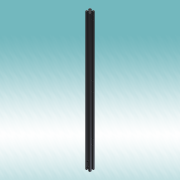
# Autodesk Inventor part: HFSB5-2020-550-LCH-RWV-AH30-BH240-CH280-DH442-EH462
Saved by Autodesk Inventor 2015 (Build 190159000, 159)
## iProperties
Category: PARTsolutions
Company: MISUMI
Created: 2016-02-28
Part Number: HFSB5-2020-550-LCH-RWV-AH30-BH240-CH280-DH442-EH462
Catalog Web Link: www.cadenas.de
Description: NFS5-2020, NFSB5-2020, HFS5-2020, HFSB5-2020, CAF5-2020, HFSY5-2020, NFSF5-2020, HFSF5-2020, HFSFB5-2020, NFST5-2020, HFST5-2020, HFSTB5-2020, HFSH5-2020, HFSC5-2020-HFS5 Series Aluminum Extrusions 20 Square -1 Slot-
Vendor: MISUMI
Document SubType Name: Modeling
Designer: psAdmin
Manufacturer: MISUMI
Mass: 98.1163 g
Surface Area: 954.349 cm^2
Volume: 98.1163 cm^3
Density: 1 g/cm^3
Material: 一般
Appearance: PSOLRGB-175-175-175
PSOL_IDENT_0: {$CADENAS_DATA\23d-libs\misumi\metric\38_al_extrusions_blackets\5\hfs5_2020.prj},646 {VTYP=3D},{NB=H
PSOL_IDENT_1: FSB5-2020-550-LCH-RWV-AH30-BH240-CH280-DH442-EH462},{LINA=HFSB5-2020-550-LCH-RWV-AH30-BH240-CH280-DH
PSOL_IDENT_2: 442-EH462},{NN=NFS5-2020, NFSB5-2020, HFS5-2020, HFSB5-2020, CAF5-2020, HFSY5-2020, NFSF5-2020, HFSF
PSOL_IDENT_3: 5-2020, HFSFB5-2020, NFST5-2020, HFST5-2020, HFSTB5-2020, HFSH5-2020, HFSC5-2020},{DATE=17.07.2015 1
PSOL_IDENT_4: 0:47:07},{GEOMDATE=28.10.2014 00:00:00},{VERSION=},{LINEID=140},{LINESUBID=-1},{WBVAR=L,ALT1,ALT2,AL
PSOL_IDENT_5: T4,ALT5,CP5,DL5,DR5,ALT6,ALT9,ALT10,ALT11,HP6,NHL6,DL6,NHR6,DR6,ALT7,ALT8,NH9,AH,BH,CH,DH,EH,NH10,AV
PSOL_IDENT_6: ,BV,CV,DV,EV,NH11,AP,BP,CP,DP,EP,ALT12,ALT13,Z,NH12,XA,XB,XC,XD,XE,NH13,YA,YB,YC,YD,YE,ALT16,HP16,DL
PSOL_IDENT_7: 16,DR16,ALT17,HQ17,JLP,ALT20}  {NB=HFSB5-2020-550-LCH-RWV-AH30-BH240-CH280-DH442-EH462},{LINA=HFSB5-
PSOL_IDENT_8: 2020-550-LCH-RWV-AH30-BH240-CH280-DH442-EH462},{KT=DUMMY},{PN=HFSB5-2020-550-LCH-RWV-AH30-BH240-CH28
PSOL_IDENT_9: 0-DH442-EH462},{TPS=HFSB5-2020},{MAT=A6N01SS-T5 Aluminum Alloy or 6005A-T5 Aluminum Alloy},{ST=Black
PSOL_IDENT_10: Anodize},{FRMW=20},{FRMH=20},{FRD=4.2},{L=550},{MASS=0.5},{SA=183},{LX=0.742x10^4},{LY=0.742x10^4},
PSOL_IDENT_11: {ALT1=},{M1=0},{DPL1=0},{DPR1=0},{ALT1PN=},{ALT2=},{ALT2ALG= '','w/o End Tapping (Heli-Coil Insert)'
PSOL_IDENT_12: ,'LHP','with LHP (Tapping on the Left (Heli-Coil Insert))','RHP','with RHP (Tapping on the Right (He
PSOL_IDENT_13: li-Coil Insert))','HPW','with HPW (Tapping on Both Ends (Heli-Coil Insert))' },{M2=0},{DP2=0},{ALT2P
PSOL_IDENT_14: N=},{ALT4=},{ALT4ALG= '', 'w/o SC (High Precision Cut)', 'SC', 'with SC (High Precision Cut)' },{ALT
PSOL_IDENT_15: 4PN=},{ALT5=},{ALT5ALG= '','w/o 45 Degree Cut','1','with 45 Degree Cut' },{CP5=},{CP5ALG= '','N/A' }
PSOL_IDENT_16: ,{DL5=},{DL5ALG= '','N/A' },{DR5=},{DR5ALG= '','N/A' },{FRMLALT5=0},{FRMRALT5=0},{ALT5PN=},{ALT6=1},
PSOL_IDENT_17: {ALT6ALG= '','w/o Fastening Location Wrench Access Hole Alterations','1','with Fastening Location Wr
PSOL_IDENT_18: ench Access Hole Alterations' },{ALT9=1},{ALT9ALG= '','w/o Location Specified Wrench Access Hole Alt
PSOL_IDENT_19: eratons (Horizontal)','1','with Location Specified Wrench Access Hole Alteratons (Horizontal)' },{AL
PSOL_IDENT_20: T10=},{ALT10ALG= '','w/o Location Specified Wrench Access Hole Alteratons (Vertical)','1','with Loca
PSOL_IDENT_21: tion Specified Wrench Access Hole Alteratons (Vertical)' },{ALT11=},{ALT11ALG= '','w/o Location Spec
PSOL_IDENT_22: ified Wrench Access Hole Alteratons (Crisscross)','1','with Location Specified Wrench Access Hole Al
PSOL_IDENT_23: teratons (Crisscross)' },{HP6=LR},{HP6ALG= 'L','Left','R','Right','LR','Both Sides' },{NHL6=C},{NHL6
PSOL_IDENT_24: ALG= 'C','C (Wrench Holes in Single Line)','W','W (Wrench Holes in Two Lines)','E','E (Wrench Holes
PSOL_IDENT_25: in Three Lines)' },{DL6=H},{DL6ALG= 'H','H (Horizontal)','V','V (Vertical)','P','P (Crisscross)' },{
PSOL_IDENT_26: NHR6=W},{NHR6ALG= 'C','C (Wrench Holes in Single Line)','W','W (Wrench Holes in Two Lines)','E','E (
PSOL_IDENT_27: Wrench Holes in Three Lines)' },{DR6=V},{DR6ALG= 'H','H (Horizontal)','V','V (Vertical)','P','P (Cri
PSOL_IDENT_28: sscross)' },{HL6=10},{HL6D=10},{HR6=10},{HR6D=10},{J6=20},{J6D=20},{K6=20},{K6D=0},{DD6=7.35},{DD6AL
PSOL_IDENT_29: G=7.35},{ALT7=},{ALT7ALG= '','w/o FL (Shifts The Wrench Hole on The Left Side 3mm Toward The Left En
PSOL_IDENT_30: d)','FL','with FL (Shifts The Wrench Hole on The Left Side 3mm Toward The Left End)' },{ALT8=},{ALT8
PSOL_IDENT_31: ALG= '','w/o FR (Shifts The Wrench Hole on The Right Side 3mm Toward The Right End)','FR','with FR (
PSOL_IDENT_32: Shifts The Wrench Hole on The Right Side 3mm Toward The Right End)' },{ALT678PN=-LCH-RWV},{NH9=5},{N
PSOL_IDENT_33: H9MAX=5},{NH9ALG=[1:5/1]},{AH=30.0},{AHMIN=7},{AHMAX=505},{AHALG=[7:505/0.5]},{BH=240.0},{BHMIN=39.5
PSOL_IDENT_34: },{BHMAX=514.5},{BHALG=[39.5:514.5/0.5]},{CH=280.0},{CHMIN=249.5},{CHMAX=524},{CHALG=[249.5:524/0.5]
PSOL_IDENT_35: },{DH=442.0},{DHMIN=289.5},{DHMAX=533.5},{DHALG=[289.5:533.5/0.5]},{EH=462.0},{EHMIN=451.5},{EHMAX=5
PSOL_IDENT_36: 43},{EHALG=[451.5:543/0.5]},{NH10=0},{NH10MAX=5},{NH10ALG=[0]},{AV=0.0},{AVMIN=7},{AVMAX=552.5},{AVA
PSOL_IDENT_37: LG=[0]},{BV=0.0},{BVMIN=9.5},{BVMAX=562},{BVALG=[0]},{CV=0.0},{CVMIN=9.5},{CVMAX=571.5},{CVALG=[0]},
PSOL_IDENT_38: {DV=0.0},{DVMIN=9.5},{DVMAX=581},{DVALG=[0]},{EV=0.0},{EVMIN=9.5},{EVMAX=543},{EVALG=[0]},{NH11=0},{
PSOL_IDENT_39: NH11MAX=5},{NH11ALG=[0]},{AP=0.0},{APMIN=7},{APMAX=552.5},{APALG=[0]},{BP=0.0},{BPMIN=9.5},{BPMAX=56
PSOL_IDENT_40: 2},{BPALG=[0]},{CP=0.0},{CPMIN=9.5},{CPMAX=571.5},{CPALG=[0]},{DP=0.0},{DPMIN=9.5},{DPMAX=581},{DPAL
PSOL_IDENT_41: G=[0]},{EP=0.0},{EPMIN=9.5},{EPMAX=543},{EPALG=[0]},{ALT9PN=-AH30-BH240-CH280-DH442-EH462},{ALT10PN=
PSOL_IDENT_42: },{ALT11PN=},{ALT91011PN=-AH30-BH240-CH280-DH442-EH462},{ALT12=},{ALT12ALG= '','w/o Counterbore Hole
PSOL_IDENT_43: in Specified Position (Vertical)','1','with Counterbore Hole in Specified Position (Vertical)' },{A
PSOL_IDENT_44: LT13=},{ALT13ALG= '','w/o Counterbore Hole in Specified Position (Horizontal)','1','with Counterbore
PSOL_IDENT_45: Hole in Specified Position (Horizontal)' },{Z=},{ZALG= '','N/A' },{DD12=0.0},{DD112=0.0},{NH12=0},{
PSOL_IDENT_46: NH12MAX=5},{NH12ALG=[0]},{XA=0.0},{XAMIN=7},{XAMAX=545},{XAALG=[0]},{XB=0.0},{XBMIN=2},{XBMAX=547},{
PSOL_IDENT_47: XBALG=[0]},{XC=0.0},{XCMIN=2},{XCMAX=549},{XCALG=[0]},{XD=0.0},{XDMIN=2},{XDMAX=551},{XDALG=[0]},{XE=
PSOL_IDENT_48: 0.0},{XEMIN=2},{XEMAX=543},{XEALG=[0]},{NH13=0},{NH13MAX=5},{NH13ALG=[0]},{YA=0.0},{YAMIN=7},{YAMAX=
PSOL_IDENT_49: 545},{YAALG=[0]},{YB=0.0},{YBMIN=2},{YBMAX=547},{YBALG=[0]},{YC=0.0},{YCMIN=2},{YCMAX=549},{YCALG=[0
PSOL_IDENT_50: ]},{YD=0.0},{YDMIN=2},{YDMAX=551},{YDALG=[0]},{YE=0.0},{YEMIN=2},{YEMAX=543},{YEALG=[0]},{ALT12PN=},
PSOL_IDENT_51: {ALT13PN=},{ALT1213PN=},{ALT16=},{ALT16ALG= '','w/o M Type Hole Alteration','1','with M Type Hole Al
PSOL_IDENT_52: teration' },{HP16=},{HP16ALG= '','N/A' },{DL16=},{DL16ALG= '','N/A' },{DR16=},{DR16ALG= '','N/A' },{
PSOL_IDENT_53: H116=0},{D16=0.0},{ALT16PN=},{ALT17=},{ALT17ALG= '','w/o L Type Hole Alteration (Top)','1','with L T
PSOL_IDENT_54: ype Hole Alteration (Top)' },{HQ17=0},{HQ17ALG=0},{JLP=0},{JLPMIN=4.9},{JLPMAX=0},{JLPALG=[0]},{L17=
PSOL_IDENT_55: 0},{D17=0.0},{ALT17PN=},{ALT20=},{ALT20PN=},{ERRORALT01=OK},{ERRORALT02=OK},{ERRORALT05=OK},{ERRORAL
PSOL_IDENT_56: T06091=OK},{ERRORALT06092=OK},{ERRORALT06093=OK},{ERRORALT06094=OK},{ERRORALT06101=OK},{ERRORALT0610
PSOL_IDENT_57: 2=OK},{ERRORALT06103=OK},{ERRORALT06104=OK},{ERRORALT06111=OK},{ERRORALT06112=OK},{ERRORALT06113=OK}
PSOL_IDENT_58: ,{ERRORALT06114=OK},{ERRORALT06121=OK},{ERRORALT06122=OK},{ERRORALT06123=OK},{ERRORALT06124=OK},{ERR
PSOL_IDENT_59: ORALT06131=OK},{ERRORALT06132=OK},{ERRORALT06133=OK},{ERRORALT06134=OK},{ERRORALT0616=OK},{ERRORALT0
PSOL_IDENT_60: 6171=OK},{ERRORALT06172=OK},{ERRORALT06173=OK},{ERRORALT0911=OK},{ERRORALT0913=OK},{ERRORALT0916=OK}
PSOL_IDENT_61: ,{ERRORALT0917=OK},{ERRORALT1011=OK},{ERRORALT1012=OK},{ERRORALT1016=OK},{ERRORALT1017=OK},{ERRORALT
PSOL_IDENT_62: 1112=OK},{ERRORALT1113=OK},{ERRORALT1116=OK},{ERRORALT1117=OK},{ERRORALT1216=OK},{ERRORALT1217=OK},{
PSOL_IDENT_63: ERRORALT1316=OK},{ERRORALT1317=OK},{ERRORALT1617=OK},{ERRORPN=},{TFW=0}
NN: NFS5-2020, NFSB5-2020, HFS5-2020, HFSB5-2020, CAF5-2020, HFSY5-2020, NFSF5-2020, HFSF5-2020, HFSFB5-2020, NFST5-2020, HFST5-2020, HFSTB5-2020, HFSH5-2020, HFSC5-2020
NT: HFS5 Series Aluminum Extrusions 20 Square -1 Slot-
NB: HFSB5-2020-550-LCH-RWV-AH30-BH240-CH280-DH442-EH462
NBSYN: $PN.
LINA: HFSB5-2020-550-LCH-RWV-AH30-BH240-CH280-DH442-EH462
PN: HFSB5-2020-550-LCH-RWV-AH30-BH240-CH280-DH442-EH462
TPS: HFSB5-2020
MAT: A6N01SS-T5 Aluminum Alloy or 6005A-T5 Aluminum Alloy
ST: Black Anodize
L: 550
MASS: 0.5
SA: 183
LX: 0.742x10^4
LY: 0.742x10^4
ALT1: w/o End Tapping
M1: 0
DPL1: 0
DPR1: 0
ALT2: w/o End Tapping (Heli-Coil Insert)
M2: 0
DP2: 0
ALT4: w/o SC (High Precision Cut)
ALT5: w/o 45 Degree Cut
CP5: N/A
DL5: N/A
DR5: N/A
ALT6: with Fastening Location Wrench Access Hole Alterations
ALT9: with Location Specified Wrench Access Hole Alteratons (Horizontal)
ALT10: w/o Location Specified Wrench Access Hole Alteratons (Vertical)
ALT11: w/o Location Specified Wrench Access Hole Alteratons (Crisscross)
HP6: Both Sides
NHL6: C (Wrench Holes in Single Line)
DL6: H (Horizontal)
NHR6: W (Wrench Holes in Two Lines)
DR6: V (Vertical)
HL6D: 10
HR6D: 10
J6D: 20
K6D: 0
DD6: 7.35
ALT7: w/o FL (Shifts The Wrench Hole on The Left Side 3mm Toward The Left End)
ALT8: w/o FR (Shifts The Wrench Hole on The Right Side 3mm Toward The Right End)
NH9: 5
AH: 30.0
BH: 240.0
CH: 280.0
DH: 442.0
EH: 462.0
NH10: 0
AV: 0.0
BV: 0.0
CV: 0.0
DV: 0.0
EV: 0.0
NH11: 0
AP: 0.0
BP: 0.0
CP: 0.0
DP: 0.0
EP: 0.0
ALT12: w/o Counterbore Hole in Specified Position (Vertical)
ALT13: w/o Counterbore Hole in Specified Position (Horizontal)
Z: N/A
DD12: 0.0
DD112: 0.0
NH12: 0
XA: 0.0
XB: 0.0
XC: 0.0
XD: 0.0
XE: 0.0
NH13: 0
YA: 0.0
YB: 0.0
YC: 0.0
YD: 0.0
YE: 0.0
ALT16: w/o M Type Hole Alteration
HP16: N/A
DL16: N/A
DR16: N/A
H116: 0
D16: 0.0
ALT17: w/o L Type Hole Alteration (Top)
HQ17: 0
JLP: 0
D17: 0.0
ALT20: w/o CW (End Face C Chamfering)
SUPPLIER: MISUMI
ARTICLENO: HFSB5-2020-550-LCH-RWV-AH30-BH240-CH280-DH442-EH462
BOMINFO: HFSB5-2020-550-LCH-RWV-AH30-BH240-CH280-DH442-EH462
CREATOR: CADENAS GmbH
Title: HFSB5-2020-550-LCH-RWV-AH30-BH240-CH280-DH442-EH462
Author: Cadenas PARTsolutions
Comments: HFS5 Series Aluminum Extrusions 20 Square -1 Slot-
Autodesk Inventor part; units mm, degrees
sketch "Sketch_1" plane through (0, 0, 0) normal (0, 0, 1) x (1, 0, 0)
  line L0 (-10, 3) -> (-8, 3)
  line L1 (-8, 3) -> (-8, 6)
  line L2 (-8, 6) -> (-7.0607, 6)
  line L3 (-7.0607, 6) -> (-4, 2.9393)
  line L4 (-4, 2.9393) -> (-4, 0.5196)
  line L5 (-4, 0.5196) -> (-3.7, 0)
  line L6 (-3.7, 0) -> (-4, -0.5196)
  line L7 (-4, -0.5196) -> (-4, -2.9393)
  line L8 (-4, -2.9393) -> (-7.0607, -6)
  line L9 (-7.0607, -6) -> (-8, -6)
  line L10 (-8, -6) -> (-8, -3)
  line L11 (-8, -3) -> (-10, -3)
  line L12 (-10, -3) -> (-10, -9)
  arc A0 (-10, -9) -> (-9, -10) centre (-9, -9) ccw
  line L13 (-9, -10) -> (-3, -10)
  line L14 (-3, -10) -> (-3, -8)
  line L15 (-3, -8) -> (-6, -8)
  line L16 (-6, -8) -> (-6, -7.0607)
  line L17 (-6, -7.0607) -> (-2.9393, -4)
  line L18 (-2.9393, -4) -> (-0.5196, -4)
  line L19 (-0.5196, -4) -> (0, -3.7)
  line L20 (0, -3.7) -> (0.5196, -4)
  line L21 (0.5196, -4) -> (2.9393, -4)
  line L22 (2.9393, -4) -> (6, -7.0607)
  line L23 (6, -7.0607) -> (6, -8)
  line L24 (6, -8) -> (3, -8)
  line L25 (3, -8) -> (3, -10)
  line L26 (3, -10) -> (9, -10)
  arc A1 (9, -10) -> (10, -9) centre (9, -9) ccw
  line L27 (10, -9) -> (10, -3)
  line L28 (10, -3) -> (8, -3)
  line L29 (8, -3) -> (8, -6)
  line L30 (8, -6) -> (7.0607, -6)
  line L31 (7.0607, -6) -> (4, -2.9393)
  line L32 (4, -2.9393) -> (4, -0.5196)
  line L33 (4, -0.5196) -> (3.7, 0)
  line L34 (3.7, 0) -> (4, 0.5196)
  line L35 (4, 0.5196) -> (4, 2.9393)
  line L36 (4, 2.9393) -> (7.0607, 6)
  line L37 (7.0607, 6) -> (8, 6)
  line L38 (8, 6) -> (8, 3)
  line L39 (8, 3) -> (10, 3)
  line L40 (10, 3) -> (10, 9)
  arc A2 (10, 9) -> (9, 10) centre (9, 9) ccw
  line L41 (9, 10) -> (3, 10)
  line L42 (3, 10) -> (3, 8)
  line L43 (3, 8) -> (6, 8)
  line L44 (6, 8) -> (6, 7.0607)
  line L45 (6, 7.0607) -> (2.9393, 4)
  line L46 (2.9393, 4) -> (0.5196, 4)
  line L47 (0.5196, 4) -> (0, 3.7)
  line L48 (0, 3.7) -> (-0.5196, 4)
  line L49 (-0.5196, 4) -> (-2.9393, 4)
  line L50 (-2.9393, 4) -> (-6, 7.0607)
  line L51 (-6, 7.0607) -> (-6, 8)
  line L52 (-6, 8) -> (-3, 8)
  line L53 (-3, 8) -> (-3, 10)
  line L54 (-3, 10) -> (-9, 10)
  arc A3 (-9, 10) -> (-10, 9) centre (-9, 9) ccw
  line L55 (-10, 9) -> (-10, 3)
  constraints: 112 end point, 8 point on circle, 4 centre point
extrude "Extrusion1" add sketch "Sketch_1" against normal blind 550
sketch "Sketch2" plane through (0, 0, -550) normal (0, 0, -1) x (-1, 0, 0)
  point P0 (0, 0)
hole "Hole1" at (0, 0, -550) direction (0, 0, 1) diameter 4.2 depth 550
sketch "Sketch_13" plane through (0, 0, 0) normal (0, 1, 0) x (1, 0, 0)
  line L0 (10, 10) -> (-10, 10)
  line L1 (-10, 10) -> (-10, 13.675)
  line L2 (-10, 13.675) -> (10, 13.675)
  line L3 (10, 13.675) -> (10, 10)
  line L4 (10, 10) -> (-10, 10)
  constraints: 10 end point
revolve "Revolution1" cut sketch "Sketch_13" angle 360 about axis through (10, 0, -10) along (1, 0, 0)
sketch "Sketch_22" plane through (0, 0, 0) normal (1, 0, 0) x (0, 0, -1)
  line L0 (540, -10) -> (540, 10)
  line L1 (540, 10) -> (543.675, 10)
  line L2 (543.675, 10) -> (543.675, -10)
  line L3 (543.675, -10) -> (540, -10)
  line L4 (540, -10) -> (540, 10)
  constraints: 10 end point
revolve "Revolution2" cut sketch "Sketch_22" angle 360 about axis through (0, -10, -540) along (0, -1, 0)
sketch "Sketch_23" plane through (0, 0, 0) normal (1, 0, 0) x (0, 0, -1)
  line L0 (520, -10) -> (520, 10)
  line L1 (520, 10) -> (523.675, 10)
  line L2 (523.675, 10) -> (523.675, -10)
  line L3 (523.675, -10) -> (520, -10)
  line L4 (520, -10) -> (520, 10)
  constraints: 10 end point
revolve "Revolution3" cut sketch "Sketch_23" angle 360 about axis through (0, -10, -520) along (0, -1, 0)
sketch "Sketch_62" plane through (0, 0, 0) normal (0, 1, 0) x (1, 0, 0)
  line L0 (10, 30) -> (-10, 30)
  line L1 (-10, 30) -> (-10, 33.675)
  line L2 (-10, 33.675) -> (10, 33.675)
  line L3 (10, 33.675) -> (10, 30)
  line L4 (10, 30) -> (-10, 30)
  constraints: 10 end point
revolve "Revolution4" cut sketch "Sketch_62" angle 360 about axis through (10, 0, -30) along (1, 0, 0)
sketch "Sketch_25" plane through (0, 0, 0) normal (0, 1, 0) x (1, 0, 0)
  line L0 (10, 240) -> (-10, 240)
  line L1 (-10, 240) -> (-10, 243.675)
  line L2 (-10, 243.675) -> (10, 243.675)
  line L3 (10, 243.675) -> (10, 240)
  line L4 (10, 240) -> (-10, 240)
  constraints: 10 end point
revolve "Revolution5" cut sketch "Sketch_25" angle 360 about axis through (10, 0, -240) along (1, 0, 0)
sketch "Sketch_26" plane through (0, 0, 0) normal (0, 1, 0) x (1, 0, 0)
  line L0 (10, 280) -> (-10, 280)
  line L1 (-10, 280) -> (-10, 283.675)
  line L2 (-10, 283.675) -> (10, 283.675)
  line L3 (10, 283.675) -> (10, 280)
  line L4 (10, 280) -> (-10, 280)
  constraints: 10 end point
revolve "Revolution6" cut sketch "Sketch_26" angle 360 about axis through (10, 0, -280) along (1, 0, 0)
sketch "Sketch_27" plane through (0, 0, 0) normal (0, 1, 0) x (1, 0, 0)
  line L0 (10, 442) -> (-10, 442)
  line L1 (-10, 442) -> (-10, 445.675)
  line L2 (-10, 445.675) -> (10, 445.675)
  line L3 (10, 445.675) -> (10, 442)
  line L4 (10, 442) -> (-10, 442)
  constraints: 10 end point
revolve "Revolution7" cut sketch "Sketch_27" angle 360 about axis through (10, 0, -442) along (1, 0, 0)
sketch "Sketch_28" plane through (0, 0, 0) normal (0, 1, 0) x (1, 0, 0)
  line L0 (10, 462) -> (-10, 462)
  line L1 (-10, 462) -> (-10, 465.675)
  line L2 (-10, 465.675) -> (10, 465.675)
  line L3 (10, 465.675) -> (10, 462)
  line L4 (10, 462) -> (-10, 462)
  constraints: 10 end point
revolve "Revolution8" cut sketch "Sketch_28" angle 360 about axis through (10, 0, -462) along (1, 0, 0)
ref_plane "C1_XY" through (0, 0, 0) normal (0, 0, 1) x (1, 0, 0)
ref_plane "C1_YZ" through (0, 0, 0) normal (1, 0, 0) x (0, 1, 0)
ref_plane "C1_ZX" through (0, 0, 0) normal (0, 1, 0) x (0, 0, 1)
body "Solid1"
